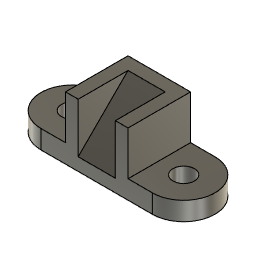
A2 (Autodesk Fusion 360 design; units mm, degrees)
Autodesk Fusion 360 part; units mm, degrees
sketch "base" plane through (0, 0, 0) normal (0, 0, 1) x (1, 0, 0)
  line L0 (89, 32) -> (-89, 32)
  line L1 (-89, 32) -> (-89, -32)
  line L2 (-89, -32) -> (89, -32)
  line L3 (89, -32) -> (89, 32)
  line L4 (89, 32) -> (-89, -32) construction
  line L5 (-89, 32) -> (89, -32) construction
  dimension "d1" = 178
  dimension "d2" = 64
  constraint horizontal L0
  constraint perpendicular L0 L1
  constraint parallel L0 L2
  constraint parallel L1 L3
  constraint coincident L4 origin
  constraint coincident L5 origin
  measures "d1" distance of L1.end L2.end
  measures "d2" distance of L0.end L1.end
extrude "Extrude1" add sketch "base" along normal blind 19
fillet "Fillet1" radius 32 4 edges at (89, -32, 9.5) (89, 32, 9.5) (-89, -32, 9.5) (-89, 32, 9.5)
sketch "circles" plane through (0, 0, 19) normal (0, 0, 1) x (-1, 0, 0)
  arc A0 (57, -32) -> (57, 32) centre (57, 0) ccw
  line L0 (57, 32) -> (-57, 32)
  arc A1 (-57, 32) -> (-57, -32) centre (-57, 0) ccw
  line L1 (-57, -32) -> (57, -32)
  line L2 (57, 32) -> (57, -32) construction
  line L3 (-57, 32) -> (-57, -32) construction
  circle A2 centre (-57, 0) radius 11
  circle A3 centre (57, 0) radius 11
  dimension "d6" = 64
  dimension "d7" = 64
  dimension "d8" = 22
  dimension "d9" = 22
  constraint vertical L2
  constraint coincident A0.end L0.start
  constraint coincident L0.end A1.start
  constraint perpendicular L0 L3
  constraint concentric A1 A2
  constraint concentric A0 A3
  measures "d6" distance of A0.end A0.start
  measures "d7" distance of L0.end A1.end
  measures "d8" diameter of A2
  measures "d9" diameter of A3
extrude "Extrude2" cut sketch "circles" against normal blind 50 contours A2 | A3
sketch "base square" plane through (0, 0, 19) normal (0, 0, 1) x (-1, 0, 0)
  circle A0 centre (57, 0) radius 11
  circle A1 centre (-57, 0) radius 11
  arc A2 (57, -32) -> (57, 32) centre (57, 0) ccw
  line L0 (57, 32) -> (-57, 32)
  arc A3 (-57, 32) -> (-57, -32) centre (-57, 0) ccw
  line L1 (-57, -32) -> (57, -32)
  line L2 (-32, -32) -> (32, -32)
  line L3 (32, -32) -> (32, 32)
  line L4 (32, 32) -> (-32, 32)
  line L5 (-32, 32) -> (-32, -32)
  line L6 (-32, -32) -> (32, 32) construction
  line L7 (32, -32) -> (-32, 32) construction
  dimension "d12" = 64
  dimension "d13" = 64
  constraint horizontal L2
  constraint perpendicular L2 L3
  constraint parallel L2 L4
  constraint parallel L3 L5
  constraint coincident L6 origin
  constraint coincident L7 origin
  measures "d12" distance of L3.end L4.end
  measures "d13" distance of L2.end L3.end
extrude "Extrude3" add sketch "base square" along normal blind 45 contours L0 L1 L2 L3 L4 L5
sketch "top rectangle" plane through (0, 0, 64) normal (0, 0, 1) x (-1, 0, 0)
  line L0 (-32, 32) -> (-32, -32)
  line L1 (-32, -32) -> (32, -32)
  line L2 (32, -32) -> (32, 32)
  line L3 (32, 32) -> (-32, 32)
  line L4 (19, 32) -> (-19, 32)
  line L5 (-19, 32) -> (-19, -19)
  line L6 (-19, -19) -> (19, -19)
  line L7 (19, -19) -> (19, 32)
  dimension "d16" = 13
  dimension "d17" = 38
  dimension "d18" = 51
  constraint horizontal L4
  constraint vertical L5
  constraint horizontal L6
  constraint vertical L7
  measures "d16" distance of L2.end L4.start
  measures "d17" distance of L4.start L4.end
  measures "d18" distance of L4.start L6.end
extrude "Extrude4" cut sketch "top rectangle" against normal blind 51 contours L3 L4 L5 L6 L7
sketch "Sketch6" plane through (-19, 0, 0) normal (1, 0, 0) x (0, 1, 0)
  line L0 (19, 64) -> (-32, 64)
  line L1 (-32, 64) -> (-32, 13)
  line L2 (-32, 13) -> (19, 13)
  line L3 (19, 13) -> (19, 64)
  line L4 (-32, 13) -> (19, 13)
  line L5 (19, 13) -> (19, 64)
  line L6 (-32, 13) -> (19, 64)
  constraint coincident L1.end L2.start
  constraint coincident L2.end L3.start
  constraint coincident L0.start L3.end
extrude "Extrude5" add sketch "Sketch6" along normal blind 38 contours L2 L3 L4 L5 L6
equation "d1 = 114 mm + 32 mm + 32 mm"
equation "d14 = 64 mm - 19 mm"
equation "d19 = -64 mm + 19 mm - 6 mm"
named bodies: "A2"
